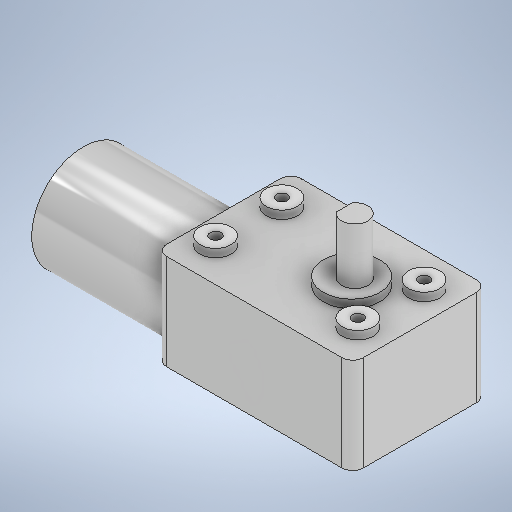
# Autodesk Inventor part: motor
Saved by Autodesk Inventor 2025.2 (Build 292293000, 293)
## iProperties
Created: 2025-04-14
Part Number: motor
Material: Generic
Document SubType Name: Modeling
Designer: 3lin2
Density: 1 g/cm^3
Appearance: Default
Author: 3lin2
Autodesk Inventor part; units mm, degrees
ref_plane "YZ Plane" through (0, 0, 0) normal (1, 0, 0) x (0, 1, 0)
ref_plane "XZ Plane" through (0, 0, 0) normal (0, 1, 0) x (-1, 0, 0)
ref_plane "XY Plane" through (0, 0, 0) normal (0, 0, 1) x (1, 0, 0)
sketch "Sketch1" plane through (0, 0, 0) normal (0, 1, 0) x (-1, 0, 0)
  line L0 (22.987, 15.748) -> (-22.987, 15.748)
  line L1 (-22.987, 15.748) -> (-22.987, -15.748)
  line L2 (-22.987, -15.748) -> (22.987, -15.748)
  line L3 (22.987, -15.748) -> (22.987, 15.748)
  point P0 (0, 0)
  dimension "d0" = 45.974
  dimension "d1" = 31.496
  dimension "d2" = 22.987
  dimension "d3" = 15.748
  constraints: 8 end point, 2 parallel, 1 horizontal, 1 perpendicular
  measures "d0" distance of L2.end L1.end
  measures "d1" distance of L1.end L0.end
  measures "d2" distance from line of point (0, 0) L3
  measures "d3" distance from line of L2 point (0, 0)
extrude "Extrusion1" add sketch "Sketch1" along normal blind 22.352
sketch "Sketch2" plane through (-22.987, 0, -15.748) normal (-1, 0, 0) x (0, 0, 1)
  circle A0 centre (17.78, 9.017) radius 12.065
  line L0 (0, 0) -> (0, 22.352) projected
  line L1 (0, 22.352) -> (31.496, 22.352) projected
  point P0 (15.748, 0)
  dimension "d6" = 24.13
  dimension "d7" = 17.78
  dimension "d8" = 13.335
  constraints: 1 centre point
  measures "d6" diameter of A0
  measures "d7" distance from line of A0.centre L0
  measures "d8" distance from line of L1 A0.centre
extrude "Extrusion2" add sketch "Sketch2" along normal blind 30.734
sketch "Sketch3" plane through (0, 22.352, 0) normal (0, 1, 0) x (1, 0, 0)
  circle A0 centre (7.747, 0) radius 3.048
  line L0 (22.987, -15.748) -> (22.987, 15.748) projected
  line L1 (-22.987, 15.748) -> (-22.987, -15.748) projected
  point P0 (0, 0)
  dimension "d11" = 6.096
  dimension "d12" = 15.24
  constraints: 1 centre point
  measures "d11" diameter of A0
  measures "d12" distance from line of A0.centre L0
extrude "Extrusion3" add sketch "Sketch3" along normal blind 14.986
fillet "Fillet1" radius 2.54 4 edges at (22.987, 11.176, 15.748) (22.987, 11.176, -15.748) (-22.987, 11.176, 15.748) (-22.987, 11.176, -15.748)
sketch "Sketch4" plane through (7.747, 37.338, 0) normal (0, 1, 0) x (1, 0, 0)
  circle A0 centre (0, 0) radius 3.048 projected
  line L0 (-2.4384, 1.8288) -> (-2.4384, -1.8288)
  arc A1 (-2.4384, 1.8288) -> (-2.4384, -1.8288) centre (0, 0) ccw
  point P0 (-7.747, 0)
  dimension "d16" = 0.6096
  constraints: 4 point on circle, 2 end point, 1 centre point, 1 concentric, 1 vertical
  measures "d16" distance edge to line of A0 L0
extrude "Extrusion4" cut sketch "Sketch4" against normal blind 14.986 contours L0 A0 picked at (-2.5495, -0.4226)
sketch "Sketch6" plane through (0, 22.352, 0) normal (0, 1, 0) x (1, 0, 0)
  circle A0 centre (16.1925, 7.7597) radius 3.6195
  circle A1 centre (16.1925, -7.747) radius 3.6195
  circle A2 centre (-17.0815, -7.747) radius 3.6195
  circle A3 centre (-17.0815, 7.7597) radius 3.6195
  line L0 (20.447, 15.748) -> (-20.447, 15.748) projected
  line L1 (-20.447, -15.748) -> (20.447, -15.748) projected
  line L2 (22.987, -13.208) -> (22.987, 13.208) projected
  point P0 (0, 0)
  dimension "d22" = 7.239
  dimension "d23" = 7.239
  dimension "d24" = 7.239
  dimension "d25" = 7.239
  dimension "d26" = 7.9883
  dimension "d27" = 8.001
  dimension "d28" = 0
  dimension "d29" = 0
  dimension "d30" = 0
  dimension "d31" = 6.7945
  dimension "d32" = 33.274
  dimension "d33" = 0
  constraints: 4 centre point
  measures "d22" diameter of A0
  measures "d23" diameter of A1
  measures "d24" diameter of A2
  measures "d25" diameter of A3
  measures "d26" distance from line of A0.centre L0
  measures "d27" distance from line of L1 A1.centre
  measures "d28" vertical distance of A1.centre A2.centre
  measures "d29" vertical distance of A0.centre A3.centre
  measures "d30" horizontal distance of A1.centre A0.centre
  measures "d31" distance from line of A1.centre L2
  measures "d32" distance of A2.centre A1.centre
  measures "d33" horizontal distance of A2.centre A3.centre
extrude "Extrusion5" add sketch "Sketch6" along normal blind 1.905
sketch "Sketch8" plane through (16.1925, 24.257, -7.7597) normal (0, 1, 0) x (1, 0, 0)
  circle A0 centre (0, 0) radius 1.27
  point P0 (-16.1925, -7.7597)
  dimension "d36" = 2.54
  constraints: 1 centre point
  measures "d36" diameter of A0
sketch "Sketch9" plane through (16.1925, 24.257, 7.747) normal (0, 1, 0) x (1, 0, 0)
  circle A0 centre (0, 0) radius 1.27
  point P0 (-16.1925, 7.747)
  dimension "d37" = 2.54
  constraints: 1 centre point
  measures "d37" diameter of A0
sketch "Sketch10" plane through (-17.0815, 24.257, -7.7597) normal (0, 1, 0) x (1, 0, 0)
  circle A0 centre (0, 0) radius 1.27
  point P0 (17.0815, -7.7597)
  dimension "d38" = 2.54
  constraints: 1 centre point
  measures "d38" diameter of A0
sketch "Sketch11" plane through (-17.0815, 24.257, 7.747) normal (0, 1, 0) x (1, 0, 0)
  circle A0 centre (0, 0) radius 1.27
  point P0 (17.0815, 7.747)
  dimension "d39" = 2.54
  constraints: 1 centre point
  measures "d39" diameter of A0
extrude "Extrusion6" cut sketch "Sketch11" against normal blind 2.54
extrude "Extrusion7" cut sketch "Sketch10" against normal blind 2.54
extrude "Extrusion8" cut sketch "Sketch8" against normal blind 2.54
extrude "Extrusion9" cut sketch "Sketch9" against normal blind 2.54
sketch "Sketch12" plane through (0, 22.352, 0) normal (0, 1, 0) x (1, 0, 0)
  circle A0 centre (6.985, 0) radius 6.604
  line L0 (22.987, -13.208) -> (22.987, 13.208) projected
  point P0 (0, 0)
  dimension "d48" = 13.208
  dimension "d49" = 16.002
  constraints: 1 centre point
  measures "d48" diameter of A0
  measures "d49" distance from line of A0.centre L0
extrude "Extrusion10" add sketch "Sketch12" along normal blind 1.905
body "Solid1"
